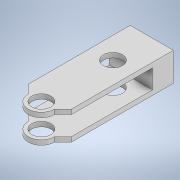
# Autodesk Inventor part: Joint1
Saved by Autodesk Inventor 2022.3 (Build 263350000, 350)
## iProperties
Created: 2022-05-28
Part Number: Joint1
Material: Generic
Document SubType Name: Modeling
Designer: Mlees
Density: 1 g/cm^3
Appearance: Default
Author: Mlees
Autodesk Inventor part; units mm, degrees
ref_plane "YZ Plane" through (0, 0, 0) normal (1, 0, 0) x (0, 1, 0)
ref_plane "XZ Plane" through (0, 0, 0) normal (0, 1, 0) x (-1, 0, 0)
ref_plane "XY Plane" through (0, 0, 0) normal (0, 0, 1) x (1, 0, 0)
sketch "Sketch1" plane through (0, 0, 0) normal (0, 1, 0) x (-1, 0, 0)
  circle A0 centre (0, 0) radius 8
  arc A1 (11, 0) -> (-11, 0) centre (0, 0) ccw
  line L0 (-11, 0) -> (-18.0711, -7.0711)
  line L1 (-11, 0) -> (-1, 0) construction
  line L2 (-18.0711, -7.0711) -> (-18.0711, -32.4711)
  line L3 (11, 0) -> (18.0711, -7.0711)
  line L4 (11, 0) -> (21, 0) construction
  line L5 (18.0711, -7.0711) -> (18.0711, -32.4711)
  line L6 (18.0711, -32.4711) -> (-18.0711, -32.4711)
  dimension "d0" = 16
  dimension "d2" = 10
  dimension "d3" = 135
  dimension "d4" = 25.4
  dimension "d5" = 10
  dimension "d6" = 45
  constraints: 14 end point, 2 centre point, 2 coincident, 2 equal length, 2 horizontal, 2 point on circle, 2 vertical, 1 perpendicular
  measures "d0" diameter of A0
  measures "d2" distance of L0.start L0.end
  measures "d3" angle of L0 L1
  measures "d4" distance of L0.end L2.end
  measures "d5" distance of L3.start L3.end
  measures "d6" angle of L3 L4
extrude "Extrusion1" add sketch "Sketch1" along normal blind 24
sketch "Sketch2" plane through (18.0711, 0, -32.4711) normal (0, 0, -1) x (-1, 0, 0)
  line L0 (7.0711, 0) -> (0, 0) projected
  line L1 (0, 24) -> (36.1421, 24) projected
  line L2 (0, 0) -> (36.1421, 0)
  line L3 (36.1421, 0) -> (36.1421, 24)
  line L4 (36.1421, 24) -> (0, 24)
  line L5 (0, 24) -> (0, 0)
  point P0 (18.0711, 0)
  constraints: 8 end point, 2 parallel, 1 horizontal, 1 perpendicular
extrude "Extrusion2" add sketch "Sketch2" along normal blind 60
sketch "Sketch3" plane through (18.0711, 0, -7.0711) normal (1, 0, 0) x (0, 0, -1)
  line L0 (-7.0711, 0) -> (-7.0711, 24) projected
  line L1 (52.9289, 12) -> (52.9289, 20)
  line L2 (52.9289, 12) -> (52.9289, 4)
  line L3 (52.9289, 4) -> (-7.0711, 4)
  line L4 (-7.0711, 4) -> (-7.0711, 20)
  line L5 (-7.0711, 20) -> (52.9289, 20)
  line L6 (-18.0711, 0) -> (-18.0711, 24) projected
  line L7 (-7.0711, 20) -> (-18.0711, 20)
  line L8 (-18.0711, 20) -> (-18.0711, 4)
  line L9 (-18.0711, 4) -> (-7.0711, 4)
  line L10 (-7.0711, 4) -> (-7.0711, 20)
  line L11 (67.9289, 12) -> (67.9289, 20)
  line L12 (67.9289, 20) -> (52.9289, 20)
  line L13 (67.9289, 12) -> (67.9289, 4)
  line L14 (67.9289, 4) -> (52.9289, 4)
  dimension "d13" = 8
  constraints: 26 end point, 5 perpendicular, 4 point on line, 2 parallel, 1 horizontal, 1 vertical
  measures "d13" distance of L1.start L2.end
extrude "Extrusion3" cut sketch "Sketch3" against normal through all
sketch "Sketch4" plane through (0, 24, 0) normal (0, 1, 0) x (1, 0, 0)
  circle A0 centre (0, 60) radius 8
  point P0 (0, 0)
  dimension "d18" = 16
  constraints: 1 centre point
  measures "d18" diameter of A0
extrude "Extrusion4" cut sketch "Sketch4" against normal through all
body "Solid1"
